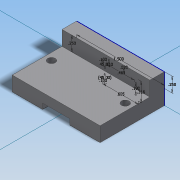
# Autodesk Inventor part: xt-60 holder
Saved by Autodesk Inventor 2014 SP2 (Build 180246200, 246)
## iProperties
Created: 2014-06-06
Part Number: xt-60 holder
Material: Generic
Document SubType Name: Modeling
Designer: dliu
Density: 1 g/cm^3
Appearance: Default
Author: dliu
Autodesk Inventor part; units mm, degrees
ref_plane "YZ Plane" through (0, 0, 0) normal (1, 0, 0) x (0, 1, 0)
ref_plane "XZ Plane" through (0, 0, 0) normal (0, 1, 0) x (-1, 0, 0)
ref_plane "XY Plane" through (0, 0, 0) normal (0, 0, 1) x (1, 0, 0)
sketch "XT60" plane through (0, 0, 0) normal (0, 0, 1) x (1, 0, 0)
  line L0 (-7.6835, 4.0132) -> (7.6835, 4.0132) construction
  line L1 (7.6835, 4.0132) -> (7.6835, -4.0132)
  line L2 (7.6835, -4.0132) -> (-7.6835, -4.0132) construction
  line L3 (-7.6835, -4.0132) -> (-7.6835, 4.0132) construction
  line L4 (-7.6835, 4.0132) -> (7.6835, -4.0132) construction
  line L5 (7.6835, 4.0132) -> (-7.6835, -4.0132) construction
  line L6 (-7.6835, 2.2171) -> (-5.8874, 4.0132)
  line L7 (-7.6835, 2.2171) -> (-5.1435, 2.2171) construction
  line L8 (-10.7569, 0) -> (10.7569, 0) projected
  line L9 (-7.6835, -2.2171) -> (-5.8874, -4.0132)
  line L10 (-7.6835, -2.2171) -> (-5.1435, -2.2171) construction
  line L11 (-7.6835, -2.2171) -> (-7.6835, 2.2171)
  line L12 (-5.8874, 4.0132) -> (7.6835, 4.0132)
  line L13 (7.6835, -4.0132) -> (-5.8874, -4.0132)
  point P0 (0, 0)
  dimension "d0" = 15.367
  dimension "d1" = 8.0264
  dimension "d2" = 2.54
  dimension "d3" = 45
  dimension "d4" = 2.54
  dimension "d5" = 45
  constraints: 26 end point, 4 point on line, 3 collinear, 3 horizontal, 2 equal length, 2 midpoint, 2 parallel, 2 perpendicular
  measures "d0" distance of L1.end L2.end
  measures "d1" distance of L0.end L1.end
  measures "d2" distance of L6.start L6.end
  measures "d3" angle of L7 L6
  measures "d4" distance of L9.start L9.end
  measures "d5" angle of L9 L10
sketch "Sketch2" plane through (0, 0, 0) normal (0, 0, 1) x (1, 0, 0)
  line L0 (-7.6835, 2.2171) -> (-5.8874, 4.0132) projected
  line L1 (-5.8874, 4.0132) -> (7.6835, 4.0132) projected
  line L2 (-7.6835, -2.2171) -> (-7.6835, 2.2171) projected
  line L3 (-7.6835, -2.2171) -> (-5.8874, -4.0132) projected
  line L4 (7.6835, -4.0132) -> (-5.8874, -4.0132) projected
  line L5 (7.6835, 4.0132) -> (7.6835, -4.0132) projected
  line L6 (8.1915, 4.5212) -> (-6.0979, 4.5212)
  line L7 (-6.0979, 4.5212) -> (-8.1915, 2.4276)
  line L8 (-8.1915, 2.4276) -> (-8.1915, -2.4276)
  line L9 (-8.1915, -2.4276) -> (-6.0979, -4.5212)
  line L10 (-6.0979, -4.5212) -> (8.1915, -4.5212)
  line L11 (8.1915, -4.5212) -> (8.1915, 4.5212)
  line L12 (7.4295, 3.7592) -> (-5.7822, 3.7592)
  line L13 (-5.7822, 3.7592) -> (-7.4295, 2.1119)
  line L14 (-7.4295, 2.1119) -> (-7.4295, -2.1119)
  line L15 (-7.4295, -2.1119) -> (-5.7822, -3.7592)
  line L16 (-5.7822, -3.7592) -> (7.4295, -3.7592)
  line L17 (7.4295, -3.7592) -> (7.4295, 3.7592)
  line L18 (-19.05, 6.35) -> (19.05, 6.35)
  line L19 (19.05, 6.35) -> (19.05, 0)
  line L20 (19.05, 0) -> (-19.05, 0)
  line L21 (-19.05, 0) -> (-19.05, 6.35)
  line L22 (-5.9055, -2.413) -> (5.9055, -2.413)
  line L23 (5.9055, -2.413) -> (5.9055, 2.413)
  line L24 (5.9055, 2.413) -> (-5.9055, 2.413)
  line L25 (-5.9055, 2.413) -> (-5.9055, -2.413)
  line L26 (-5.9055, -2.413) -> (5.9055, 2.413) construction
  line L27 (5.9055, -2.413) -> (-5.9055, 2.413) construction
  line L28 (-19.05, 6.35) -> (19.05, 6.35)
  line L29 (19.05, 6.35) -> (19.05, 12.7)
  line L30 (19.05, 12.7) -> (-19.05, 12.7)
  line L31 (-19.05, 12.7) -> (-19.05, 6.35)
  point P0 (0, 0)
  dimension "d6" = 0.254
  dimension "d7" = 0.508
  dimension "d8" = 38.1
  dimension "d9" = 6.35
  dimension "d25" = 11.811
  dimension "d26" = 4.826
  dimension "d29" = 6.35
  constraints: 52 end point, 6 parallel, 4 midpoint, 3 horizontal, 3 perpendicular, 10 other
  measures "d6" distance between parallel lines of L12 L1
  measures "d7" distance between parallel lines of L6 L1
  measures "d8" distance of L18.start L18.end
  measures "d9" distance between parallel lines of L20 L18
  measures "d25" distance of L24.end L23.end
  measures "d26" distance of L23.end L22.end
  measures "d29" distance of L18.end L29.end
extrude "Extrusion1" add sketch "Sketch2" along normal blind 27.94 contours L2 L20 L8 L7 L6 L11 L5 L1 L0 | L0 L1 L5 L20 L17 L12 L13 L14 L2 | L14 L13 L12 L17 L20 L23 L24 L25 | L20 L21 L18 L19 L11 L6 L7 L8 | L25 L24 L23 L20
extrude "Extrusion2" cut sketch "Sketch2" along normal blind 18.3896 contours L20 L25 L22 L23 L17 L16 L15 L14 | L14 L13 L12 L17 L20 L23 L24 L25 | L25 L24 L23 L20 | L20 L23 L22 L25
extrude "Extrusion3" cut sketch "Sketch2" along normal blind 10.6172 contours L2 L20 L8 L7 L6 L11 L5 L1 L0 | L0 L1 L5 L20 L17 L12 L13 L14 L2 | L20 L14 L15 L16 L17 L5 L4 L3 L2 | L2 L3 L4 L5 L20 L11 L10 L9 L8 | L20 L25 L22 L23 L17 L16 L15 L14 | L14 L13 L12 L17 L20 L23 L24 L25 | L25 L24 L23 L20 | L20 L23 L22 L25
sketch "Sketch3" plane through (0, 0, 0) normal (0, 1, 0) x (-1, 0, 0)
  point P0 (-16.002, 13.97)
  point P1 (0, 0)
  dimension "d16" = 16.002
  dimension "d17" = 13.97
  measures "d16" horizontal distance of point (0, 0) point (-16.002, 13.97)
  measures "d17" vertical distance of point (0, 0) point (-16.002, 13.97)
hole "Hole1" at (16.002, 0, 13.97) direction (0, 1, 0) diameter 3.2766 end through all clearance for "Oval Head Machine Screw" size "#4" standard "Ansi Unified Screw Threads"
mirror "Mirror1" about plane through (0, 0, 0) normal (1, 0, 0) of "Hole1"
extrude "Extrusion4" cut sketch "Sketch2" along normal through all contours L25 L24 L23 L20 | L20 L23 L22 L25
extrude "Extrusion5" add sketch "Sketch2" along normal blind 6.35 contours L31 L30 L29 L18
body "Solid1"
